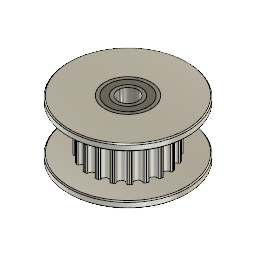
GT2 20-Tooth Idler Pulley (Autodesk Fusion 360 design; units mm, degrees)
Autodesk Fusion 360 part; units mm, degrees
sketch "Sketch1" plane through (0, 0, 0) normal (0, 0, 1) x (1, 0, 0)
  circle A0 centre (0, 0) radius 9
  circle A1 centre (0, 0) radius 5.9
  circle A2 centre (0, 0) radius 3.5
  circle A3 centre (0, 0) radius 3
  circle A4 centre (0, 0) radius 1.5
  circle A5 centre (0, 0) radius 2
  arc A6 (0.9502, 5.8157) -> (0.7519, 5.8447) centre (0, 0) ccw
  arc A7 (2.5212, 5.3263) -> (2.3386, 5.4089) centre (0, 0) ccw
  arc A8 (1.0703, 5.6267) -> (2.1354, 5.3146) centre (1.6041, 5.4748) ccw
  arc A9 (1.0703, 5.6267) -> (0.9502, 5.8157) centre (0.926, 5.6677) ccw
  arc A10 (2.3386, 5.4089) -> (2.1354, 5.3146) centre (2.279, 5.2713) ccw
  arc A11 (-0.7209, 5.682) -> (0.3886, 5.7144) centre (-0.1662, 5.7026) ccw
  arc A12 (0.5527, 5.8669) -> (0.3886, 5.7144) centre (0.5386, 5.7175) ccw
  arc A13 (0.7519, 5.8447) -> (0.5527, 5.8669) centre (0, 0) ccw
  arc A14 (-0.8935, 5.8247) -> (-1.0911, 5.791) centre (0, 0) ccw
  arc A15 (-0.7209, 5.682) -> (-0.8935, 5.8247) centre (-0.8707, 5.6764) ccw
  arc A16 (-2.4414, 5.1812) -> (-1.3962, 5.5548) centre (-1.9203, 5.3721) ccw
  arc A17 (-1.2873, 5.7505) -> (-1.3962, 5.5548) centre (-1.2546, 5.6041) ccw
  arc A18 (-1.0911, 5.791) -> (-1.2873, 5.7505) centre (0, 0) ccw
  arc A19 (-2.6497, 5.2635) -> (-2.8272, 5.1704) centre (0, 0) ccw
  arc A20 (-2.4414, 5.1812) -> (-2.6497, 5.2635) centre (-2.5823, 5.1295) ccw
  arc A21 (-3.923, 4.1731) -> (-3.0444, 4.8514) centre (-3.4864, 4.5158) ccw
  arc A22 (-3.0013, 5.0712) -> (-3.0444, 4.8514) centre (-2.925, 4.9422) ccw
  arc A23 (-2.8272, 5.1704) -> (-3.0013, 5.0712) centre (0, 0) ccw
  arc A24 (-4.1465, 4.1871) -> (-4.2865, 4.0437) centre (0, 0) ccw
  arc A25 (-3.923, 4.1731) -> (-4.1465, 4.1871) centre (-4.041, 4.0805) ccw
  arc A26 (-5.0206, 2.7566) -> (-4.3946, 3.6732) centre (-4.7112, 3.2174) ccw
  arc A27 (-4.4215, 3.8956) -> (-4.3946, 3.6732) centre (-4.309, 3.7964) ccw
  arc A28 (-4.2865, 4.0437) -> (-4.4215, 3.8956) centre (0, 0) ccw
  arc A29 (-5.2375, 2.7008) -> (-5.3263, 2.5212) centre (0, 0) ccw
  arc A30 (-5.0206, 2.7566) -> (-5.2375, 2.7008) centre (-5.1042, 2.6321) ccw
  arc A31 (-5.6267, 1.0703) -> (-5.3146, 2.1354) centre (-5.4749, 1.6041) ccw
  arc A32 (-5.4089, 2.3386) -> (-5.3146, 2.1354) centre (-5.2713, 2.279) ccw
  arc A33 (-5.3263, 2.5212) -> (-5.4089, 2.3386) centre (0, 0) ccw
  arc A34 (-5.8157, 0.9502) -> (-5.8447, 0.7519) centre (0, 0) ccw
  arc A35 (-5.6267, 1.0703) -> (-5.8157, 0.9502) centre (-5.6677, 0.926) ccw
  arc A36 (-5.682, -0.7209) -> (-5.7144, 0.3886) centre (-5.7026, -0.1662) ccw
  arc A37 (-5.8669, 0.5527) -> (-5.7144, 0.3886) centre (-5.7175, 0.5386) ccw
  arc A38 (-5.8447, 0.7518) -> (-5.8669, 0.5527) centre (0, 0) ccw
  arc A39 (-5.8247, -0.8935) -> (-5.791, -1.0911) centre (0, 0) ccw
  arc A40 (-5.682, -0.7209) -> (-5.8247, -0.8935) centre (-5.6764, -0.8708) ccw
  arc A41 (-5.1812, -2.4414) -> (-5.5548, -1.3962) centre (-5.3721, -1.9203) ccw
  arc A42 (-5.7505, -1.2873) -> (-5.5548, -1.3962) centre (-5.6041, -1.2546) ccw
  arc A43 (-5.791, -1.0911) -> (-5.7505, -1.2873) centre (0, 0) ccw
  arc A44 (-5.2635, -2.6497) -> (-5.1704, -2.8272) centre (0, 0) ccw
  arc A45 (-5.1812, -2.4414) -> (-5.2635, -2.6497) centre (-5.1295, -2.5823) ccw
  arc A46 (-4.1731, -3.923) -> (-4.8514, -3.0444) centre (-4.5158, -3.4864) ccw
  arc A47 (-5.0712, -3.0013) -> (-4.8514, -3.0444) centre (-4.9422, -2.925) ccw
  arc A48 (-5.1704, -2.8272) -> (-5.0712, -3.0013) centre (0, 0) ccw
  arc A49 (-4.1871, -4.1465) -> (-4.0437, -4.2865) centre (0, 0) ccw
  arc A50 (-4.1731, -3.923) -> (-4.1871, -4.1465) centre (-4.0805, -4.041) ccw
  arc A51 (-2.7566, -5.0206) -> (-3.6732, -4.3946) centre (-3.2174, -4.7112) ccw
  arc A52 (-3.8956, -4.4215) -> (-3.6732, -4.3946) centre (-3.7964, -4.309) ccw
  arc A53 (-4.0437, -4.2865) -> (-3.8956, -4.4215) centre (0, 0) ccw
  arc A54 (-2.7008, -5.2375) -> (-2.5212, -5.3263) centre (0, 0) ccw
  arc A55 (-2.7566, -5.0206) -> (-2.7008, -5.2375) centre (-2.6321, -5.1042) ccw
  arc A56 (-1.0703, -5.6267) -> (-2.1354, -5.3146) centre (-1.6041, -5.4749) ccw
  arc A57 (-2.3386, -5.4089) -> (-2.1354, -5.3146) centre (-2.279, -5.2713) ccw
  arc A58 (-2.5212, -5.3263) -> (-2.3386, -5.4089) centre (0, 0) ccw
  arc A59 (-0.9502, -5.8157) -> (-0.7519, -5.8447) centre (0, 0) ccw
  arc A60 (-1.0703, -5.6267) -> (-0.9502, -5.8157) centre (-0.926, -5.6677) ccw
  arc A61 (0.7209, -5.682) -> (-0.3886, -5.7144) centre (0.1662, -5.7026) ccw
  arc A62 (-0.5527, -5.8669) -> (-0.3886, -5.7144) centre (-0.5386, -5.7175) ccw
  arc A63 (-0.7518, -5.8447) -> (-0.5527, -5.8669) centre (0, 0) ccw
  arc A64 (0.8935, -5.8247) -> (1.0911, -5.791) centre (0, 0) ccw
  arc A65 (0.7209, -5.682) -> (0.8935, -5.8247) centre (0.8708, -5.6764) ccw
  arc A66 (2.4414, -5.1812) -> (1.3962, -5.5548) centre (1.9203, -5.3721) ccw
  arc A67 (1.2873, -5.7505) -> (1.3962, -5.5548) centre (1.2546, -5.6041) ccw
  arc A68 (1.0911, -5.791) -> (1.2873, -5.7505) centre (0, 0) ccw
  arc A69 (2.6497, -5.2635) -> (2.8272, -5.1704) centre (0, 0) ccw
  arc A70 (2.4414, -5.1812) -> (2.6497, -5.2635) centre (2.5823, -5.1295) ccw
  arc A71 (3.923, -4.1731) -> (3.0444, -4.8514) centre (3.4864, -4.5158) ccw
  arc A72 (3.0013, -5.0712) -> (3.0444, -4.8514) centre (2.925, -4.9422) ccw
  arc A73 (2.8272, -5.1704) -> (3.0013, -5.0712) centre (0, 0) ccw
  arc A74 (4.1465, -4.1871) -> (4.2865, -4.0437) centre (0, 0) ccw
  arc A75 (3.923, -4.1731) -> (4.1465, -4.1871) centre (4.041, -4.0805) ccw
  arc A76 (5.0206, -2.7566) -> (4.3946, -3.6732) centre (4.7112, -3.2174) ccw
  arc A77 (4.4215, -3.8956) -> (4.3946, -3.6732) centre (4.309, -3.7964) ccw
  arc A78 (4.2865, -4.0437) -> (4.4215, -3.8956) centre (0, 0) ccw
  arc A79 (5.2375, -2.7008) -> (5.3263, -2.5212) centre (0, 0) ccw
  arc A80 (5.0206, -2.7566) -> (5.2375, -2.7008) centre (5.1042, -2.6321) ccw
  arc A81 (5.6267, -1.0703) -> (5.3146, -2.1354) centre (5.4749, -1.6041) ccw
  arc A82 (5.4089, -2.3386) -> (5.3146, -2.1354) centre (5.2713, -2.279) ccw
  arc A83 (5.3263, -2.5212) -> (5.4089, -2.3386) centre (0, 0) ccw
  arc A84 (5.8157, -0.9502) -> (5.8447, -0.7519) centre (0, 0) ccw
  arc A85 (5.6267, -1.0703) -> (5.8157, -0.9502) centre (5.6677, -0.926) ccw
  arc A86 (5.682, 0.7209) -> (5.7144, -0.3886) centre (5.7026, 0.1662) ccw
  arc A87 (5.8669, -0.5527) -> (5.7144, -0.3886) centre (5.7175, -0.5386) ccw
  arc A88 (5.8447, -0.7518) -> (5.8669, -0.5527) centre (0, 0) ccw
  arc A89 (5.8247, 0.8935) -> (5.791, 1.0911) centre (0, 0) ccw
  arc A90 (5.682, 0.7209) -> (5.8247, 0.8935) centre (5.6764, 0.8708) ccw
  arc A91 (5.1812, 2.4414) -> (5.5548, 1.3962) centre (5.3721, 1.9203) ccw
  arc A92 (5.7505, 1.2873) -> (5.5548, 1.3962) centre (5.6041, 1.2546) ccw
  arc A93 (5.791, 1.0911) -> (5.7505, 1.2873) centre (0, 0) ccw
  arc A94 (5.2635, 2.6497) -> (5.1704, 2.8272) centre (0, 0) ccw
  arc A95 (5.1812, 2.4414) -> (5.2635, 2.6497) centre (5.1295, 2.5823) ccw
  arc A96 (4.1731, 3.923) -> (4.8514, 3.0444) centre (4.5158, 3.4864) ccw
  arc A97 (5.0712, 3.0013) -> (4.8514, 3.0444) centre (4.9422, 2.925) ccw
  arc A98 (5.1704, 2.8272) -> (5.0712, 3.0013) centre (0, 0) ccw
  arc A99 (4.1871, 4.1465) -> (4.0437, 4.2865) centre (0, 0) ccw
  arc A100 (4.1731, 3.923) -> (4.1871, 4.1465) centre (4.0805, 4.041) ccw
  arc A101 (2.7566, 5.0206) -> (3.6732, 4.3946) centre (3.2174, 4.7112) ccw
  arc A102 (3.8956, 4.4215) -> (3.6732, 4.3946) centre (3.7964, 4.309) ccw
  arc A103 (4.0437, 4.2865) -> (3.8956, 4.4215) centre (0, 0) ccw
  arc A104 (2.7008, 5.2375) -> (2.5212, 5.3263) centre (0, 0) ccw
  arc A105 (2.7566, 5.0206) -> (2.7008, 5.2375) centre (2.6321, 5.1042) ccw
  line L0 (2.279, 5.2713) -> (2.6321, 5.1042) construction
  line L1 (2.5212, 5.3263) -> (0, 0) construction
  circle A106 centre (0, 0) radius 5.15 construction
  point P0 (2.4556, 5.1877)
  point P1 (1.448, 4.9422)
  dimension "d1" = 18
  dimension "d2" = 11.8
  dimension "d3" = 7
  dimension "d11" = 0.5
  dimension "d12" = 0.5
  dimension "d13" = 3
  dimension "d24" = 0.555
  dimension "d27" = 0.15
  dimension "d30" = 360
  dimension "d31" = 0.75
  constraint coincident A0.centre A1.centre
  constraint concentric A0 A1
  constraint concentric A0 A2
  constraint concentric A1 A3
  constraint concentric A3 A4
  constraint concentric A3 A5
  constraint equal A6 A7
  constraint tangent A6 A9
  constraint tangent A8 A9
  constraint tangent A8 A10
  constraint tangent A7 A10
  constraint equal A9 A10
  constraint coincident A6.end A13.start
  constraint coincident A10.centre L0.start
  constraint coincident A105.centre L0.end
  constraint midpoint L0 P0
  constraint coincident P0 L1
  constraint midpoint A8 P1
  constraint coincident A106 P1
  measures "d1" diameter of A0
  measures "d2" diameter of A1
  measures "d3" diameter of A2
  measures "d11" distance of A4 A5
  measures "d12" distance of A2 A3
  measures "d13" diameter of A4
  measures "d24" radius of A8
  measures "d27" radius of A9
  measures "d31" distance of A1 A106
extrude "Extrude4" add sketch "Sketch1" along normal blind 8.5 contours A6 A7 A8 A9 A10 A11 A12 A13 A14 A15 A16 A17 A18 A19 A20 A21 A22 A23 A24 A25 A26 A27 A28 A29 A30 A31 A32 A33 A34 A35 A36 A37 A38 A39 A40 A41 A42 A43 A44 A45 A46 A47 A48 A49 A50 A51 A52 A53 A54 A55 A56 A57 A58 A59 A60 A61 A62 A63 A64 A65 A66 A67 A68 A69 A70 A71 A72 A73 A74 A75 A76 A77 A78 A79 A80 A81 A82 A83 A84 A85 A86 A87 A88 A89 A90 A91 A92 A93 A94 A95 A96 A97 A98 A99 A100 A101 A102 A103 A104 A105 makes body 1
extrude "Extrude5" add sketch "Sketch1" along normal blind 1 contours A0 | A1 bodies 1
extrude "Extrude6" add sketch "Sketch1" against normal blind 1 from surface at 8.5 contours A0 | A1 bodies 1
copy_body "Body->Comp2" bodies 1 removing the originals makes body 2 in component "Pulley"
extrude "Extrude1" add sketch "Sketch1" along normal up to surface (8.5 mm away) separate body contours A2 | A5 makes body 3 at (3.4956, -0.1745, 5.6667) makes body 4 at (1.9975, -0.0997, 5.6667) in component "Bearing"
extrude "Extrude2" add sketch "Sketch1" along normal up to surface (8.5 mm away) separate body contours A3 makes body 5 in component "Bearing"
chamfer "Chamfer1" distance 0.15 angle 45 4 edges at (-8.3909, 3.2545, 8.5) (-8.3909, 3.2545, 7.5) (-8.3909, -3.2545, 1) (-8.3909, -3.2545, 0) on bodies 2 in component "Pulley"
component "Pulley" placed x (1, 0, 0) y (0, 1, 0) z (0, 0, 1) at (0, 0, 0)
component "Bearing" placed x (1, 0, 0) y (0, 1, 0) z (0, 0, 1) at (0, 0, 0)
